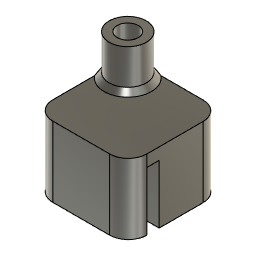
Mod - Bowden Tube Holder (Autodesk Fusion 360 design; units mm, degrees)
Autodesk Fusion 360 part; units mm, degrees
sketch "Main" plane through (0, 0, 0) normal (0, 0, 1) x (1, 0, 0) in component "Bowden Clip"
  line L0 (-13.0366, 0) -> (16.1033, 0)
  line L1 (-13.4598, -2.45) -> (15.2511, -2.45)
  line L2 (15, -2.45) -> (15, 8.75)
  circle A0 centre (0, 8.75) radius 0.875
  circle A1 centre (0, 8.75) radius 2.1
  circle A2 centre (0, 8.75) radius 1.5
  line L3 (0, -6.15) -> (11.3, -6.15)
  line L4 (0, 20.1585) -> (0, -19.1006) construction
  line L5 (-3.7, 8.75) -> (-3.7, -2.45)
  arc A3 (-3.7, -2.45) -> (0, -6.15) centre (0, -2.45) ccw
  arc A4 (11.3, -6.15) -> (15, -2.45) centre (11.3, -2.45) ccw
  circle A5 centre (0, 8.75) radius 3.7
  line L6 (11.3, 12.45) -> (0, 12.45)
  arc A6 (15, 8.75) -> (11.3, 12.45) centre (11.3, 8.75) ccw
  dimension "d1" = 2.45
  dimension "d2" = 1.75
  dimension "d3" = 4.2
  dimension "d4" = 8.75
  dimension "d5" = 15
  dimension "d6" = 3
  dimension "d7" = 3.7
  dimension "d9" = 3.7
  dimension "d11" = 3.7
  dimension "d12" = 3.7
  dimension "d14" = 3.7
  dimension "d15" = 7.4
  constraint horizontal L0
  constraint coincident origin L0
  constraint horizontal L1
  constraint perpendicular L0 L2
  constraint concentric A0 A1
  constraint vertical origin A0.centre
  constraint concentric A1 A2
  constraint horizontal L3
  constraint perpendicular L3 L4
  constraint coincident origin L4
  constraint perpendicular L3 L5
  constraint tangent L5 A3
  constraint tangent L3 A3
  constraint tangent L3 A4
  constraint tangent L2 A4
  constraint concentric A0 A5
  constraint coincident A5 L6.end
  constraint tangent A5 L6
  constraint tangent L6 A6
  constraint tangent L2 A6
  constraint horizontal L6
  measures "d1" distance of L0 L1
  measures "d2" diameter of A0
  measures "d3" diameter of A1
  measures "d4" distance of L0 A0.centre
  measures "d5" distance of L2 A0.centre
  measures "d6" diameter of A2
  measures "d7" distance of L1 L3
  measures "d9" distance of A0.centre L5
  measures "d11" radius of A3
  measures "d12" radius of A4
  measures "d14" radius of A6
  measures "d15" diameter of A5
extrude "Extrude1" add sketch "Main" along normal blind 14 contours L0 L2 L5 A5 L6 A6 | L0 L1 L2 L5 | A5 | L1 L3 A3 A4 in component "Bowden Clip"
extrude "Extrude2" add sketch "Main" along normal blind 1 contours A1 in component "Bowden Clip"
extrude "Extrude3" cut sketch "Main" along normal blind 12 contours L0 L1 L2 L5 in component "Bowden Clip"
sketch "Angle" plane through (0, 0, 0) normal (0, -1, 0) x (1, 0, 0) in component "Bowden Clip"
  line L0 (-3.7, 0) -> (15, 0)
  line L1 (15, 0) -> (15, 12)
  line L2 (-3.7, 12) -> (-3.7, 0)
  line L3 (-5.7721, 0.626) -> (17.5, 13)
  line L4 (0, 0) -> (11.3, 0)
  line L5 (15, 12) -> (-3.7, 12)
  dimension "d22" = 28
  measures "d22" angle of L3 L4
extrude "Extrude4" add sketch "Angle" along normal up to surface (2.45 mm away) contours L1 L2 L3 L5 in component "Bowden Clip"
chamfer "Chamfer1" distance 0.5 angle 45 1 edges at (-1.9579, 9.5094, 1) in component "Bowden Clip"
extrude "Extrude5" add sketch "Main" along normal blind 22 contours A5 in component "Bowden Clip"
chamfer "Chamfer2" distance 1 angle 45 1 edges at (2.6163, 6.1337, 14) in component "Bowden Clip"
sketch "Nut" plane through (0, 0, 0) normal (0, -1, 0) x (1, 0, 0) in component "Bowden Clip"
  circle A0 centre (7.7152, 5.3692) radius 1.95
  line L0 (11.2152, 11.411) -> (11.2152, -0.6726)
  line L1 (4.2328, 11.4212) -> (14.6975, 5.3794)
  line L2 (0.7328, 5.3794) -> (11.1975, 11.4212)
  line L3 (4.2152, -0.6726) -> (4.2152, 11.411)
  line L4 (-3.7, 0) -> (15, 0)
  dimension "d31" = 3.9
  dimension "d34" = 3.5
  dimension "d36" = 180
  constraint vertical L0
  measures "d31" diameter of A0
  measures "d34" distance of A0.centre L0
extrude "Extrude6" cut sketch "Nut" against normal up to surface (12.45 mm away) contours A0 in component "Bowden Clip"
extrude "Extrude7" cut sketch "Nut" against normal blind 4 in component "Bowden Clip"
extrude "Extrude8" add sketch "Nut" against normal blind 0.8 in component "Bowden Clip"
sketch "Countersink" plane through (0, 12.45, 0) normal (0, 1, 0) x (-1, 0, 0) in component "Bowden Clip"
  circle A0 centre (-7.7152, 5.3692) radius 1.95
  line L0 (-11.3, 0) -> (0, 0)
  line L1 (0, 0) -> (0, 15)
  spline S0 degree 2 poles (-2.8983, 14) (-1.2766, 15) (0, 15) knots 0 0 0 0.309625 0.309625 0.309625 weights 1 1.065427 1
  line L2 (-2.8983, 14) -> (-11.3, 14)
  line L3 (-11.3, 14) -> (-11.3, 0)
  circle A1 centre (-7.7152, 5.3692) radius 3.5
  dimension "d41" = 7
  constraint concentric A0 A1
  measures "d41" diameter of A1
extrude "Extrude9" cut sketch "Countersink" against normal blind 2.5 contours A1 in component "Bowden Clip"
component "Bowden Clip" placed x (1, 0, 0) y (0, 1, 0) z (0, 0, 1) at (0, 0, 0)
equation "d7 = d8"
equation "d8 = ( d3 / 2 ) + 1.6 mm"
equation "d9 = d8"
equation "d11 = d8"
equation "d12 = d8"
equation "d14 = d9"
equation "d15 = d3 + 3.2 mm"
named bodies: "Bowden Clip"
